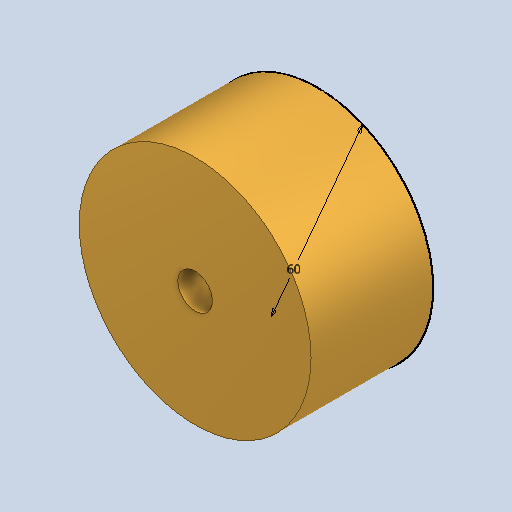
# Autodesk Inventor part: CapstonAxis0_Weights
Saved by Autodesk Inventor 2024 (Build 280153000, 153)
## iProperties
Created: 2022-10-27
Part Number: CapstonAxis0_Weights
Material: Messing, weicher Gelbton
Document SubType Name: Modeling
Designer: alexw
Density: 8.47 g/cm^3
Appearance: Messing - satiniert
Mass: 737.4 g
Surface Area: 123.559 cm^2
Volume: 87.0602 cm^3
Author: alexw
Autodesk Inventor part; units mm, degrees
ref_plane "YZ Plane" through (0, 0, 0) normal (1, 0, 0) x (0, 1, 0)
ref_plane "XZ Plane" through (0, 0, 0) normal (0, 1, 0) x (-1, 0, 0)
ref_plane "XY Plane" through (0, 0, 0) normal (0, 0, 1) x (1, 0, 0)
sketch "Skizze1" plane through (0, 0, 0) normal (0, 0, 1) x (1, 0, 0)
  circle A0 centre (0, 0) radius 30
  dimension "d0" = 60
  constraints: 2 coincident, 1 centre point
  measures "d0" diameter of A0
extrude "Extrusion1" add sketch "Skizze1" along normal blind 31.5
hole "Bohrung1" at (0, 0, 0) direction (0, 0, 1) diameter 9 end through all clearance for "Inbusschraube DIN EN ISO 4762" size "M8" standard "DIN"
